Autodesk Fusion 360 part; units mm, degrees
(part 3 of 7)
  line L27 (11.5064, 2.3612) -> (11.4015, 2.3397)
  arc A55 (11.049, 2.5657) -> (11.4015, 2.3397) centre (11.3412, 2.6336) ccw
  arc A56 (11.049, 2.5657) -> (10.9184, 3.0745) centre (0, 0) ccw
  arc A57 (11.1184, 3.4424) -> (10.9184, 3.0745) centre (11.2071, 3.1559) ccw
  line L28 (11.1184, 3.4424) -> (11.2206, 3.4741)
  spline S28 degree 5 poles (11.2206, 3.4741) (11.2255, 3.4756) (11.2353, 3.4787) (11.2497, 3.4838) (11.2687, 3.4912) (11.2922, 3.5015) (11.3154, 3.5123) (11.3384, 3.5237) (11.3614, 3.5352) (11.3844, 3.5469) (11.4073, 3.5588) (11.4301, 3.5708) (11.4528, 3.5832) (11.4754, 3.5958) (11.4979, 3.6088) (11.5202, 3.6221) (11.5425, 3.6356) (11.5646, 3.6494) (11.5868, 3.6633) (11.6088, 3.6774) (11.6307, 3.6917) (11.6526, 3.7062) (11.6744, 3.7209) (11.6962, 3.7358) (11.7178, 3.7508) (11.7394, 3.7661) (11.7609, 3.7815) (11.7823, 3.7972) (11.8036, 3.8129) (11.8249, 3.8289) (11.8461, 3.845) (11.8672, 3.8612) (11.8883, 3.8777) (11.9093, 3.8942) (11.9302, 3.911) (11.9511, 3.9279) (11.9719, 3.9449) (11.9926, 3.9621) (12.0132, 3.9794) (12.0338, 3.9969) (12.0543, 4.0145) (12.0748, 4.0323) (12.0951, 4.0502) (12.1154, 4.0682) (12.1357, 4.0864) (12.1558, 4.1047) (12.1759, 4.1231) (12.196, 4.1417) (12.216, 4.1604) (12.2359, 4.1793) (12.2557, 4.1982) (12.2755, 4.2173) (12.2952, 4.2365) (12.3148, 4.2559) (12.3344, 4.2753) (12.3539, 4.2949) (12.3733, 4.3147) (12.3927, 4.3345) (12.412, 4.3544) (12.4313, 4.3745) (12.4504, 4.3947) (12.4695, 4.415) (12.4886, 4.4355) (12.5076, 4.456) (12.5265, 4.4767) (12.5453, 4.4974) (12.5641, 4.5183) (12.5828, 4.5393) (12.6015, 4.5604) (12.62, 4.5816) (12.6385, 4.603) (12.6533, 4.6201) (12.6643, 4.633) (12.6717, 4.6417) (12.6754, 4.646) knots 0 0 0 0 0 0 0.01428571 0.02857143 0.04285714 0.05714286 0.07142857 0.08571429 0.1 0.11428571 0.12857143 0.14285714 0.15714286 0.17142857 0.18571429 0.2 0.21428571 0.22857143 0.24285714 0.25714286 0.27142857 0.28571429 0.3 0.31428571 0.32857143 0.34285714 0.35714286 0.37142857 0.38571429 0.4 0.41428571 0.42857143 0.44285714 0.45714286 0.47142857 0.48571429 0.5 0.51428571 0.52857143 0.54285714 0.55714286 0.57142857 0.58571429 0.6 0.61428571 0.62857143 0.64285714 0.65714286 0.67142857 0.68571429 0.7 0.71428571 0.72857143 0.74285714 0.75714286 0.77142857 0.78571429 0.8 0.81428571 0.82857143 0.84285714 0.85714286 0.87142857 0.88571429 0.9 0.91428571 0.92857143 0.94285714 0.95714286 0.97142857 0.98571429 1 1 1 1 1 1
  arc A58 (12.6754, 4.646) -> (12.4203, 5.2901) centre (0, 0) ccw
  spline S29 degree 5 poles (12.4203, 5.2901) (12.4147, 5.2907) (12.4034, 5.292) (12.3866, 5.2939) (12.3641, 5.2963) (12.336, 5.2991) (12.3079, 5.3019) (12.2798, 5.3045) (12.2518, 5.307) (12.2238, 5.3094) (12.1959, 5.3116) (12.168, 5.3137) (12.1401, 5.3157) (12.1122, 5.3176) (12.0844, 5.3193) (12.0566, 5.3209) (12.0288, 5.3224) (12.0011, 5.3237) (11.9734, 5.3249) (11.9457, 5.3259) (11.9181, 5.3269) (11.8905, 5.3277) (11.8629, 5.3283) (11.8354, 5.3288) (11.8079, 5.3292) (11.7805, 5.3295) (11.7531, 5.3296) (11.7257, 5.3295) (11.6984, 5.3294) (11.6711, 5.3291) (11.6438, 5.3286) (11.6166, 5.328) (11.5895, 5.3272) (11.5624, 5.3263) (11.5353, 5.3253) (11.5083, 5.3241) (11.4814, 5.3227) (11.4544, 5.3212) (11.4276, 5.3196) (11.4008, 5.3178) (11.374, 5.3158) (11.3473, 5.3137) (11.3206, 5.3114) (11.2941, 5.309) (11.2675, 5.3064) (11.241, 5.3036) (11.2146, 5.3006) (11.1883, 5.2975) (11.1619, 5.2942) (11.1357, 5.2908) (11.1095, 5.2872) (11.0834, 5.2833) (11.0574, 5.2793) (11.0315, 5.2751) (11.0056, 5.2706) (10.9798, 5.266) (10.9541, 5.2612) (10.9284, 5.2563) (10.9029, 5.2511) (10.8774, 5.2458) (10.852, 5.2401) (10.8267, 5.2342) (10.8016, 5.228) (10.7766, 5.2214) (10.7517, 5.2146) (10.7269, 5.2076) (10.7021, 5.2004) (10.6775, 5.1931) (10.6529, 5.1855) (10.6285, 5.1776) (10.6045, 5.169) (10.5855, 5.1614) (10.5715, 5.1552) (10.5623, 5.1508) (10.5577, 5.1486) knots -1 -1 -1 -1 -1 -1 -0.98571429 -0.97142857 -0.95714286 -0.94285714 -0.92857143 -0.91428571 -0.9 -0.88571429 -0.87142857 -0.85714286 -0.84285714 -0.82857143 -0.81428571 -0.8 -0.78571429 -0.77142857 -0.75714286 -0.74285714 -0.72857143 -0.71428571 -0.7 -0.68571429 -0.67142857 -0.65714286 -0.64285714 -0.62857143 -0.61428571 -0.6 -0.58571429 -0.57142857 -0.55714286 -0.54285714 -0.52857143 -0.51428571 -0.5 -0.48571429 -0.47142857 -0.45714286 -0.44285714 -0.42857143 -0.41428571 -0.4 -0.38571429 -0.37142857 -0.35714286 -0.34285714 -0.32857143 -0.31428571 -0.3 -0.28571429 -0.27142857 -0.25714286 -0.24285714 -0.22857143 -0.21428571 -0.2 -0.18571429 -0.17142857 -0.15714286 -0.14285714 -0.12857143 -0.11428571 -0.1 -0.08571429 -0.07142857 -0.05714286 -0.04285714 -0.02857143 -0.01428571 0 0 0 0 0 0
  line L29 (10.5577, 5.1486) -> (10.4615, 5.1017)
  arc A59 (10.0638, 5.2329) -> (10.4615, 5.1017) centre (10.33, 5.3713) ccw
  arc A60 (10.0638, 5.2329) -> (9.8107, 5.6932) centre (0, 0) ccw
  arc A61 (9.913, 6.0993) -> (9.8107, 5.6932) centre (10.0702, 5.8438) ccw
  line L30 (9.913, 6.0993) -> (10.0042, 6.1554)
  spline S30 degree 5 poles (10.0042, 6.1554) (10.0085, 6.1581) (10.0171, 6.1635) (10.0299, 6.172) (10.0465, 6.184) (10.0666, 6.1997) (10.0864, 6.216) (10.1059, 6.2327) (10.1253, 6.2496) (10.1446, 6.2666) (10.1638, 6.2838) (10.1829, 6.3012) (10.2019, 6.3188) (10.2206, 6.3367) (10.2392, 6.3548) (10.2575, 6.3732) (10.2757, 6.3919) (10.2938, 6.4107) (10.3117, 6.4297) (10.3295, 6.4489) (10.3472, 6.4682) (10.3648, 6.4877) (10.3823, 6.5073) (10.3997, 6.5271) (10.4169, 6.5471) (10.434, 6.5672) (10.4509, 6.5875) (10.4678, 6.608) (10.4846, 6.6286) (10.5012, 6.6493) (10.5177, 6.6702) (10.5342, 6.6912) (10.5505, 6.7123) (10.5667, 6.7336) (10.5828, 6.755) (10.5988, 6.7766) (10.6147, 6.7982) (10.6305, 6.82) (10.6462, 6.842) (10.6617, 6.864) (10.6772, 6.8862) (10.6926, 6.9085) (10.7079, 6.9309) (10.7231, 6.9534) (10.7382, 6.976) (10.7531, 6.9988) (10.768, 7.0216) (10.7828, 7.0446) (10.7975, 7.0677) (10.8121, 7.0909) (10.8266, 7.1142) (10.841, 7.1376) (10.8553, 7.1611) (10.8695, 7.1847) (10.8836, 7.2085) (10.8977, 7.2323) (10.9116, 7.2562) (10.9254, 7.2803) (10.9392, 7.3044) (10.9528, 7.3286) (10.9664, 7.3529) (10.9798, 7.3774) (10.9932, 7.4019) (11.0065, 7.4265) (11.0196, 7.4512) (11.0327, 7.476) (11.0457, 7.5009) (11.0586, 7.5259) (11.0714, 7.551) (11.0841, 7.5762) (11.0968, 7.6014) (11.1068, 7.6217) (11.1143, 7.637) (11.1192, 7.6472) (11.1217, 7.6523) knots 0 0 0 0 0 0 0.01428571 0.02857143 0.04285714 0.05714286 0.07142857 0.08571429 0.1 0.11428571 0.12857143 0.14285714 0.15714286 0.17142857 0.18571429 0.2 0.21428571 0.22857143 0.24285714 0.25714286 0.27142857 0.28571429 0.3 0.31428571 0.32857143 0.34285714 0.35714286 0.37142857 0.38571429 0.4 0.41428571 0.42857143 0.44285714 0.45714286 0.47142857 0.48571429 0.5 0.51428571 0.52857143 0.54285714 0.55714286 0.57142857 0.58571429 0.6 0.61428571 0.62857143 0.64285714 0.65714286 0.67142857 0.68571429 0.7 0.71428571 0.72857143 0.74285714 0.75714286 0.77142857 0.78571429 0.8 0.81428571 0.82857143 0.84285714 0.85714286 0.87142857 0.88571429 0.9 0.91428571 0.92857143 0.94285714 0.95714286 0.97142857 0.98571429 1 1 1 1 1 1
  arc A62 (11.1217, 7.6523) -> (10.7145, 8.2127) centre (0, 0) ccw
  spline S31 degree 5 poles (10.7145, 8.2127) (10.7089, 8.2119) (10.6977, 8.2103) (10.6809, 8.2079) (10.6585, 8.2047) (10.6306, 8.2005) (10.6027, 8.1962) (10.5749, 8.1917) (10.5471, 8.1872) (10.5194, 8.1825) (10.4918, 8.1777) (10.4642, 8.1728) (10.4367, 8.1678) (10.4092, 8.1627) (10.3819, 8.1574) (10.3545, 8.1521) (10.3273, 8.1466) (10.3001, 8.141) (10.2729, 8.1352) (10.2459, 8.1294) (10.2189, 8.1234) (10.192, 8.1173) (10.1651, 8.1111) (10.1383, 8.1048) (10.1116, 8.0983) (10.085, 8.0917) (10.0584, 8.085) (10.0319, 8.0782) (10.0055, 8.0712) (9.9791, 8.0641) (9.9529, 8.0569) (9.9267, 8.0495) (9.9006, 8.0421) (9.8745, 8.0344) (9.8486, 8.0267) (9.8227, 8.0188) (9.7969, 8.0108) (9.7712, 8.0027) (9.7456, 7.9944) (9.7201, 7.986) (9.6947, 7.9774) (9.6693, 7.9687) (9.6441, 7.9599) (9.6189, 7.9509) (9.5939, 7.9418) (9.5689, 7.9325) (9.5441, 7.9231) (9.5193, 7.9135) (9.4947, 7.9038) (9.4701, 7.8939) (9.4457, 7.8839) (9.4213, 7.8737) (9.3971, 7.8633) (9.3731, 7.8527) (9.3491, 7.842) (9.3253, 7.8311) (9.3015, 7.8201) (9.2779, 7.8089) (9.2544, 7.7976) (9.2311, 7.786) (9.2079, 7.7743) (9.1849, 7.7623) (9.1621, 7.75) (9.1395, 7.7374) (9.1171, 7.7246) (9.0948, 7.7116) (9.0726, 7.6985) (9.0506, 7.6853) (9.0287, 7.6719) (9.007, 7.6581) (8.9858, 7.6438) (8.9694, 7.6317) (8.9573, 7.6222) (8.9495, 7.6157) (8.9456, 7.6124) knots -1 -1 -1 -1 -1 -1 -0.98571429 -0.97142857 -0.95714286 -0.94285714 -0.92857143 -0.91428571 -0.9 -0.88571429 -0.87142857 -0.85714286 -0.84285714 -0.82857143 -0.81428571 -0.8 -0.78571429 -0.77142857 -0.75714286 -0.74285714 -0.72857143 -0.71428571 -0.7 -0.68571429 -0.67142857 -0.65714286 -0.64285714 -0.62857143 -0.61428571 -0.6 -0.58571429 -0.57142857 -0.55714286 -0.54285714 -0.52857143 -0.51428571 -0.5 -0.48571429 -0.47142857 -0.45714286 -0.44285714 -0.42857143 -0.41428571 -0.4 -0.38571429 -0.37142857 -0.35714286 -0.34285714 -0.32857143 -0.31428571 -0.3 -0.28571429 -0.27142857 -0.25714286 -0.24285714 -0.22857143 -0.21428571 -0.2 -0.18571429 -0.17142857 -0.15714286 -0.14285714 -0.12857143 -0.11428571 -0.1 -0.08571429 -0.07142857 -0.05714286 -0.04285714 -0.02857143 -0.01428571 0 0 0 0 0 0
  line L31 (8.9456, 7.6124) -> (8.8641, 7.543)
  arc A63 (8.4463, 7.5713) -> (8.8641, 7.543) centre (8.6697, 7.7715) ccw
  arc A64 (8.4463, 7.5713) -> (8.0867, 7.9542) centre (0, 0) ccw
  arc A65 (8.0847, 8.373) -> (8.0867, 7.9542) centre (8.3005, 8.1646) ccw
  line L32 (8.0847, 8.373) -> (8.1591, 8.45)
  spline S32 degree 5 poles (8.1591, 8.45) (8.1626, 8.4536) (8.1696, 8.4611) (8.1799, 8.4725) (8.1929, 8.4881) (8.2086, 8.5084) (8.2237, 8.5291) (8.2384, 8.5501) (8.253, 8.5713) (8.2675, 8.5926) (8.2818, 8.6141) (8.296, 8.6356) (8.31, 8.6574) (8.3237, 8.6793) (8.3371, 8.7015) (8.3503, 8.724) (8.3633, 8.7465) (8.3761, 8.7693) (8.3887, 8.7922) (8.4012, 8.8151) (8.4136, 8.8383) (8.4258, 8.8615) (8.4378, 8.8848) (8.4497, 8.9083) (8.4614, 8.932) (8.473, 8.9557) (8.4844, 8.9796) (8.4956, 9.0036) (8.5067, 9.0277) (8.5177, 9.052) (8.5285, 9.0763) (8.5392, 9.1007) (8.5497, 9.1253) (8.5601, 9.1499) (8.5704, 9.1746) (8.5806, 9.1995) (8.5906, 9.2244) (8.6004, 9.2495) (8.6102, 9.2746) (8.6198, 9.2998) (8.6293, 9.3252) (8.6386, 9.3506) (8.6479, 9.3761) (8.657, 9.4017) (8.6659, 9.4273) (8.6748, 9.4531) (8.6835, 9.4789) (8.6921, 9.5049) (8.7006, 9.5309) (8.709, 9.557) (8.7172, 9.5832) (8.7254, 9.6094) (8.7334, 9.6357) (8.7413, 9.6622) (8.749, 9.6887) (8.7567, 9.7152) (8.7642, 9.7419) (8.7717, 9.7686) (8.779, 9.7954) (8.7862, 9.8222) (8.7932, 9.8492) (8.8002, 9.8762) (8.807, 9.9032) (8.8138, 9.9304) (8.8204, 9.9576) (8.8269, 9.9849) (8.8333, 10.0122) (8.8396, 10.0396) (8.8457, 10.0671) (8.8518, 10.0947) (8.8577, 10.1223) (8.8624, 10.1444) (8.8659, 10.1611) (8.8681, 10.1722) (8.8693, 10.1777) knots 0 0 0 0 0 0 0.01428571 0.02857143 0.04285714 0.05714286 0.07142857 0.08571429 0.1 0.11428571 0.12857143 0.14285714 0.15714286 0.17142857 0.18571429 0.2 0.21428571 0.22857143 0.24285714 0.25714286 0.27142857 0.28571429 0.3 0.31428571 0.32857143 0.34285714 0.35714286 0.37142857 0.38571429 0.4 0.41428571 0.42857143 0.44285714 0.45714286 0.47142857 0.48571429 0.5 0.51428571 0.52857143 0.54285714 0.55714286 0.57142857 0.58571429 0.6 0.61428571 0.62857143 0.64285714 0.65714286 0.67142857 0.68571429 0.7 0.71428571 0.72857143 0.74285714 0.75714286 0.77142857 0.78571429 0.8 0.81428571 0.82857143 0.84285714 0.85714286 0.87142857 0.88571429 0.9 0.91428571 0.92857143 0.94285714 0.95714286 0.97142857 0.98571429 1 1 1 1 1 1
  arc A66 (8.8693, 10.1777) -> (8.3355, 10.6193) centre (0, 0) ccw
  spline S33 degree 5 poles (8.3355, 10.6193) (8.3303, 10.6171) (8.3198, 10.6128) (8.3041, 10.6063) (8.2832, 10.5976) (8.2572, 10.5866) (8.2313, 10.5754) (8.2054, 10.5642) (8.1797, 10.5529) (8.154, 10.5415) (8.1284, 10.53) (8.103, 10.5184) (8.0776, 10.5067) (8.0522, 10.4949) (8.027, 10.483) (8.0019, 10.471) (7.9768, 10.4589) (7.9519, 10.4467) (7.9271, 10.4344) (7.9023, 10.422) (7.8776, 10.4095) (7.8531, 10.3969) (7.8286, 10.3842) (7.8042, 10.3714) (7.78, 10.3585) (7.7558, 10.3455) (7.7317, 10.3324) (7.7078, 10.3192) (7.6839, 10.3059) (7.6602, 10.2925) (7.6365, 10.2789) (7.613, 10.2653) (7.5895, 10.2516) (7.5662, 10.2377) (7.543, 10.2238) (7.5199, 10.2097) (7.4969, 10.1955) (7.4741, 10.1813) (7.4513, 10.1669) (7.4287, 10.1524) (7.4062, 10.1378) (7.3838, 10.123) (7.3616, 10.1082) (7.3394, 10.0932) (7.3174, 10.0782) (7.2956, 10.063) (7.2738, 10.0477) (7.2522, 10.0322) (7.2308, 10.0167) (7.2094, 10.001) (7.1883, 9.9852) (7.1672, 9.9693) (7.1464, 9.9532) (7.1257, 9.937) (7.1052, 9.9207) (7.0848, 9.9042) (7.0645, 9.8876) (7.0444, 9.8709) (7.0245, 9.8541) (7.0047, 9.8371) (6.9852, 9.8199) (6.9659, 9.8026) (6.9469, 9.785) (6.9281, 9.7672) (6.9096, 9.7492) (6.8913, 9.7311) (6.8731, 9.7129) (6.855, 9.6946) (6.8371, 9.6762) (6.8196, 9.6575) (6.8026, 9.6383) (6.7896, 9.6225) (6.7804, 9.6104) (6.7744, 9.6021) (6.7714, 9.5979) knots -1 -1 -1 -1 -1 -1 -0.98571429 -0.97142857 -0.95714286 -0.94285714 -0.92857143 -0.91428571 -0.9 -0.88571429 -0.87142857 -0.85714286 -0.84285714 -0.82857143 -0.81428571 -0.8 -0.78571429 -0.77142857 -0.75714286 -0.74285714 -0.72857143 -0.71428571 -0.7 -0.68571429 -0.67142857 -0.65714286 -0.64285714 -0.62857143 -0.61428571 -0.6 -0.58571429 -0.57142857 -0.55714286 -0.54285714 -0.52857143 -0.51428571 -0.5 -0.48571429 -0.47142857 -0.45714286 -0.44285714 -0.42857143 -0.41428571 -0.4 -0.38571429 -0.37142857 -0.35714286 -0.34285714 -0.32857143 -0.31428571 -0.3 -0.28571429 -0.27142857 -0.25714286 -0.24285714 -0.22857143 -0.21428571 -0.2 -0.18571429 -0.17142857 -0.15714286 -0.14285714 -0.12857143 -0.11428571 -0.1 -0.08571429 -0.07142857 -0.05714286 -0.04285714 -0.02857143 -0.01428571 0 0 0 0 0 0
  line L33 (6.7714, 9.5979) -> (6.7097, 9.5105)
  arc A67 (6.298, 9.4339) -> (6.7097, 9.5105) centre (6.4646, 9.6834) ccw
  arc A68 (6.298, 9.4339) -> (5.8545, 9.7154) centre (0, 0) ccw
  arc A69 (5.7485, 10.1205) -> (5.8545, 9.7154) centre (6.0093, 9.9723) ccw
  line L34 (5.7485, 10.1205) -> (5.8013, 10.2136)
  spline S34 degree 5 poles (5.8013, 10.2136) (5.8038, 10.218) (5.8088, 10.2269) (5.8159, 10.2405) (5.8246, 10.259) (5.8347, 10.2825) (5.8442, 10.3063) (5.8533, 10.3303) (5.8621, 10.3545) (5.8708, 10.3787) (5.8794, 10.403) (5.8878, 10.4274) (5.8959, 10.452) (5.9037, 10.4767) (5.9112, 10.5015) (5.9184, 10.5265) (5.9254, 10.5516) (5.9321, 10.5768) (5.9387, 10.6021) (5.9451, 10.6275) (5.9513, 10.653) (5.9573, 10.6785) (5.9632, 10.7041) (5.9688, 10.7298) (5.9743, 10.7556) (5.9796, 10.7815) (5.9847, 10.8075) (5.9896, 10.8335) (5.9943, 10.8597) (5.9989, 10.8858) (6.0034, 10.9121) (6.0077, 10.9384) (6.0118, 10.9648) (6.0157, 10.9913) (6.0195, 11.0178) (6.0232, 11.0444) (6.0266, 11.071) (6.03, 11.0977) (6.0332, 11.1245) (6.0362, 11.1513) (6.0391, 11.1782) (6.0418, 11.2051) (6.0444, 11.2321) (6.0469, 11.2592) (6.0492, 11.2863) (6.0514, 11.3134) (6.0534, 11.3406) (6.0553, 11.3679) (6.057, 11.3952) (6.0587, 11.4226) (6.0601, 11.45) (6.0615, 11.4774) (6.0627, 11.5049) (6.0638, 11.5325) (6.0647, 11.5601) (6.0655, 11.5877) (6.0662, 11.6154) (6.0667, 11.6431) (6.0671, 11.6709) (6.0674, 11.6987) (6.0676, 11.7265) (6.0676, 11.7544) (6.0675, 11.7823) (6.0673, 11.8103) (6.0669, 11.8383) (6.0664, 11.8663) (6.0658, 11.8944) (6.0651, 11.9225) (6.0642, 11.9507) (6.0633, 11.9789) (6.0622, 12.0071) (6.0612, 12.0297) (6.0604, 12.0467) (6.0598, 12.058) (6.0595, 12.0637) knots 0 0 0 0 0 0 0.01428571 0.02857143 0.04285714 0.05714286 0.07142857 0.08571429 0.1 0.11428571 0.12857143 0.14285714 0.15714286 0.17142857 0.18571429 0.2 0.21428571 0.22857143 0.24285714 0.25714286 0.27142857 0.28571429 0.3 0.31428571 0.32857143 0.34285714 0.35714286 0.37142857 0.38571429 0.4 0.41428571 0.42857143 0.44285714 0.45714286 0.47142857 0.48571429 0.5 0.51428571 0.52857143 0.54285714 0.55714286 0.57142857 0.58571429 0.6 0.61428571 0.62857143 0.64285714 0.65714286 0.67142857 0.68571429 0.7 0.71428571 0.72857143 0.74285714 0.75714286 0.77142857 0.78571429 0.8 0.81428571 0.82857143 0.84285714 0.85714286 0.87142857 0.88571429 0.9 0.91428571 0.92857143 0.94285714 0.95714286 0.97142857 0.98571429 1 1 1 1 1 1
  arc A70 (6.0595, 12.0637) -> (5.4327, 12.3586) centre (0, 0) ccw
  spline S35 degree 5 poles (5.4327, 12.3586) (5.4282, 12.3552) (5.4191, 12.3484) (5.4055, 12.3382) (5.3875, 12.3246) (5.365, 12.3074) (5.3427, 12.2902) (5.3204, 12.273) (5.2983, 12.2556) (5.2763, 12.2382) (5.2544, 12.2207) (5.2326, 12.2031) (5.2109, 12.1854) (5.1893, 12.1677) (5.1678, 12.1499) (5.1465, 12.1321) (5.1252, 12.1141) (5.1041, 12.0961) (5.0831, 12.078) (5.0622, 12.0598) (5.0414, 12.0416) (5.0207, 12.0233) (5.0002, 12.0049) (4.9798, 11.9864) (4.9595, 11.9679) (4.9393, 11.9493) (4.9193, 11.9306) (4.8993, 11.9119) (4.8795, 11.893) (4.8599, 11.8741) (4.8403, 11.8551) (4.8209, 11.8361) (4.8016, 11.8169) (4.7825, 11.7977) (4.7635, 11.7784) (4.7446, 11.7591) (4.7259, 11.7396) (4.7073, 11.7201) (4.6888, 11.7005) (4.6705, 11.6809) (4.6524, 11.6611) (4.6343, 11.6413) (4.6165, 11.6214) (4.5988, 11.6014) (4.5812, 11.5813) (4.5638, 11.5612) (4.5466, 11.5409) (4.5295, 11.5206) (4.5126, 11.5002) (4.4958, 11.4797) (4.4792, 11.4592) (4.4628, 11.4385) (4.4466, 11.4178) (4.4306, 11.3969) (4.4148, 11.376) (4.3991, 11.355) (4.3836, 11.3339) (4.3683, 11.3127) (4.3532, 11.2914) (4.3383, 11.2701) (4.3236, 11.2486) (4.3093, 11.227) (4.2952, 11.2052) (4.2815, 11.1833) (4.268, 11.1613) (4.2547, 11.1392) (4.2416, 11.117) (4.2287, 11.0948) (4.2159, 11.0725) (4.2036, 11.05) (4.1919, 11.0273) (4.1833, 11.0088) (4.1773, 10.9946) (4.1736, 10.9851) (4.1718, 10.9804) knots -1 -1 -1 -1 -1 -1 -0.98571429 -0.97142857 -0.95714286 -0.94285714 -0.92857143 -0.91428571 -0.9 -0.88571429 -0.87142857 -0.85714286 -0.84285714 -0.82857143 -0.81428571 -0.8 -0.78571429 -0.77142857 -0.75714286 -0.74285714 -0.72857143 -0.71428571 -0.7 -0.68571429 -0.67142857 -0.65714286 -0.64285714 -0.62857143 -0.61428571 -0.6 -0.58571429 -0.57142857 -0.55714286 -0.54285714 -0.52857143 -0.51428571 -0.5 -0.48571429 -0.47142857 -0.45714286 -0.44285714 -0.42857143 -0.41428571 -0.4 -0.38571429 -0.37142857 -0.35714286 -0.34285714 -0.32857143 -0.31428571 -0.3 -0.28571429 -0.27142857 -0.25714286 -0.24285714 -0.22857143 -0.21428571 -0.2 -0.18571429 -0.17142857 -0.15714286 -0.14285714 -0.12857143 -0.11428571 -0.1 -0.08571429 -0.07142857 -0.05714286 -0.04285714 -0.02857143 -0.01428571 0 0 0 0 0 0
  line L35 (4.1718, 10.9804) -> (4.1338, 10.8803)
  arc A71 (3.754, 10.7038) -> (4.1338, 10.8803) centre (3.8533, 10.9869) ccw
  arc A72 (3.754, 10.7038) -> (3.2544, 10.8661) centre (0, 0) ccw
  arc A73 (3.051, 11.2321) -> (3.2544, 10.8661) centre (3.3405, 11.1535) ccw
  line L36 (3.051, 11.2321) -> (3.0791, 11.3354)
  spline S36 degree 5 poles (3.0791, 11.3354) (3.0804, 11.3403) (3.083, 11.3502) (3.0864, 11.3652) (3.0903, 11.3852) (3.0943, 11.4105) (3.0975, 11.4359) (3.1003, 11.4614) (3.1029, 11.487) (3.1053, 11.5127) (3.1075, 11.5383) (3.1096, 11.5641) (3.1113, 11.5899) (3.1128, 11.6157) (3.1139, 11.6417) (3.1146, 11.6676) (3.1151, 11.6937) (3.1154, 11.7198) (3.1154, 11.7459) (3.1153, 11.7721) (3.115, 11.7983) (3.1145, 11.8245) (3.1138, 11.8508) (3.1129, 11.8771) (3.1118, 11.9035) (3.1105, 11.9299) (3.1089, 11.9563) (3.1072, 11.9827) (3.1053, 12.0092) (3.1033, 12.0357) (3.101, 12.0622) (3.0986, 12.0888) (3.0961, 12.1154) (3.0933, 12.142) (3.0904, 12.1686) (3.0873, 12.1953) (3.0841, 12.222) (3.0806, 12.2487) (3.0771, 12.2754) (3.0733, 12.3021) (3.0695, 12.3289) (3.0654, 12.3556) (3.0612, 12.3824) (3.0569, 12.4093) (3.0524, 12.4361) (3.0477, 12.4629) (3.0429, 12.4898) (3.038, 12.5167) (3.0329, 12.5435) (3.0276, 12.5704) (3.0223, 12.5973) (3.0167, 12.6243) (3.0111, 12.6512) (3.0053, 12.6782) (2.9993, 12.7051) (2.9932, 12.7321) (2.987, 12.7591) (2.9806, 12.786) (2.9741, 12.813) (2.9675, 12.84) (2.9607, 12.8671) (2.9538, 12.8941) (2.9467, 12.9211) (2.9396, 12.9481) (2.9323, 12.9752) (2.9248, 13.0022) (2.9172, 13.0293) (2.9095, 13.0563) (2.9017, 13.0834) (2.8937, 13.1104) (2.8857, 13.1375) (2.8791, 13.1591) (2.8741, 13.1754) (2.8707, 13.1862) (2.8691, 13.1916) knots 0 0 0 0 0 0 0.01428571 0.02857143 0.04285714 0.05714286 0.07142857 0.08571429 0.1 0.11428571 0.12857143 0.14285714 0.15714286 0.17142857 0.18571429 0.2 0.21428571 0.22857143 0.24285714 0.25714286 0.27142857 0.28571429 0.3 0.31428571 0.32857143 0.34285714 0.35714286 0.37142857 0.38571429 0.4 0.41428571 0.42857143 0.44285714 0.45714286 0.47142857 0.48571429 0.5 0.51428571 0.52857143 0.54285714 0.55714286 0.57142857 0.58571429 0.6 0.61428571 0.62857143 0.64285714 0.65714286 0.67142857 0.68571429 0.7 0.71428571 0.72857143 0.74285714 0.75714286 0.77142857 0.78571429 0.8 0.81428571 0.82857143 0.84285714 0.85714286 0.87142857 0.88571429 0.9 0.91428571 0.92857143 0.94285714 0.95714286 0.97142857 0.98571429 1 1 1 1 1 1
  arc A74 (2.8691, 13.1916) -> (2.1886, 13.3214) centre (0, 0) ccw
  spline S37 degree 5 poles (2.1886, 13.3214) (2.185, 13.317) (2.1779, 13.3082) (2.1673, 13.2949) (2.1532, 13.2772) (2.1357, 13.255) (2.1184, 13.2328) (2.1011, 13.2105) (2.084, 13.1882) (2.067, 13.1658) (2.0501, 13.1434) (2.0334, 13.121) (2.0168, 13.0985) (2.0003, 13.076) (1.9839, 13.0534) (1.9677, 13.0308) (1.9515, 13.0081) (1.9356, 12.9854) (1.9197, 12.9627) (1.904, 12.9399) (1.8884, 12.917) (1.8729, 12.8942) (1.8576, 12.8712) (1.8424, 12.8483) (1.8274, 12.8253) (1.8125, 12.8022) (1.7977, 12.7792) (1.7831, 12.756) (1.7686, 12.7329) (1.7542, 12.7097) (1.74, 12.6864) (1.7259, 12.6631) (1.712, 12.6398) (1.6983, 12.6164) (1.6847, 12.593) (1.6712, 12.5696) (1.6579, 12.5461) (1.6447, 12.5226) (1.6317, 12.499) (1.6189, 12.4754) (1.6062, 12.4518) (1.5937, 12.4281) (1.5813, 12.4043) (1.5691, 12.3806) (1.5571, 12.3568) (1.5453, 12.3329) (1.5336, 12.309) (1.5221, 12.2851) (1.5108, 12.2611) (1.4997, 12.2371) (1.4887, 12.2131) (1.478, 12.189) (1.4674, 12.1649) (1.4571, 12.1407) (1.447, 12.1165) (1.437, 12.0922) (1.4273, 12.068) (1.4177, 12.0436) (1.4084, 12.0193) (1.3992, 11.9949) (1.3904, 11.9704) (1.3819, 11.9459) (1.3737, 11.9213) (1.3658, 11.8967) (1.3582, 11.872) (1.3509, 11.8473) (1.3437, 11.8226) (1.3366, 11.7979) (1.3298, 11.7731) (1.3235, 11.7483) (1.3178, 11.7233) (1.3141, 11.7032) (1.3118, 11.6881) (1.3106, 11.678) (1.31, 11.6729) knots -1 -1 -1 -1 -1 -1 -0.98571429 -0.97142857 -0.95714286 -0.94285714 -0.92857143 -0.91428571 -0.9 -0.88571429 -0.87142857 -0.85714286 -0.84285714 -0.82857143 -0.81428571 -0.8 -0.78571429 -0.77142857 -0.75714286 -0.74285714 -0.72857143 -0.71428571 -0.7 -0.68571429 -0.67142857 -0.65714286 -0.64285714 -0.62857143 -0.61428571 -0.6 -0.58571429 -0.57142857 -0.55714286 -0.54285714 -0.52857143 -0.51428571 -0.5 -0.48571429 -0.47142857 -0.45714286 -0.44285714 -0.42857143 -0.41428571 -0.4 -0.38571429 -0.37142857 -0.35714286 -0.34285714 -0.32857143 -0.31428571 -0.3 -0.28571429 -0.27142857 -0.25714286 -0.24285714 -0.22857143 -0.21428571 -0.2 -0.18571429 -0.17142857 -0.15714286 -0.14285714 -0.12857143 -0.11428571 -0.1 -0.08571429 -0.07142857 -0.05714286 -0.04285714 -0.02857143 -0.01428571 0 0 0 0 0 0
  line L37 (1.31, 11.6729) -> (1.2981, 11.5665)
  arc A75 (0.9742, 11.3011) -> (1.2981, 11.5665) centre (0.9999, 11.6) ccw
  arc A76 (0.9742, 11.3011) -> (0.4499, 11.3341) centre (0, 0) ccw
  arc A77 (0.1618, 11.638) -> (0.4499, 11.3341) centre (0.4618, 11.6338) ccw
  line L38 (0.1618, 11.638) -> (0.1633, 11.745)
  spline S38 degree 5 poles (0.1633, 11.745) (0.1634, 11.7501) (0.1634, 11.7603) (0.1631, 11.7757) (0.1619, 11.796) (0.1594, 11.8215) (0.1562, 11.8469) (0.1526, 11.8724) (0.1487, 11.8978) (0.1447, 11.9232) (0.1404, 11.9487) (0.136, 11.9741) (0.1313, 11.9995) (0.1263, 12.0249) (0.1209, 12.0503) (0.1151, 12.0757) (0.1091, 12.101) (0.1029, 12.1264) (0.0965, 12.1517) (0.0899, 12.177) (0.083, 12.2023) (0.076, 12.2276) (0.0688, 12.2529) (0.0614, 12.2781) (0.0537, 12.3034) (0.0459, 12.3286) (0.0378, 12.3538) (0.0296, 12.379) (0.0212, 12.4042) (0.0126, 12.4293) (0.0039, 12.4545) (-0.0051, 12.4796) (-0.0142, 12.5047) (-0.0235, 12.5298) (-0.0329, 12.5549) (-0.0425, 12.5799) (-0.0523, 12.605) (-0.0623, 12.63) (-0.0724, 12.655) (-0.0826, 12.6799) (-0.093, 12.7049) (-0.1036, 12.7298) (-0.1143, 12.7547) (-0.1252, 12.7796) (-0.1363, 12.8045) (-0.1474, 12.8293) (-0.1588, 12.8541) (-0.1702, 12.8789) (-0.1819, 12.9037) (-0.1936, 12.9285) (-0.2055, 12.9532) (-0.2176, 12.9779) (-0.2298, 13.0026) (-0.2421, 13.0272) (-0.2546, 13.0519) (-0.2672, 13.0765) (-0.2799, 13.101) (-0.2928, 13.1256) (-0.3058, 13.1501) (-0.3189, 13.1746) (-0.3322, 13.1991) (-0.3456, 13.2236) (-0.3592, 13.248) (-0.3729, 13.2724) (-0.3867, 13.2967) (-0.4006, 13.3211) (-0.4147, 13.3454) (-0.4288, 13.3697) (-0.4432, 13.3939) (-0.4576, 13.4182) (-0.4722, 13.4424) (-0.4839, 13.4617) (-0.4928, 13.4762) (-0.4987, 13.4858) (-0.5017, 13.4907) knots 0 0 0 0 0 0 0.01428571 0.02857143 0.04285714 0.05714286 0.07142857 0.08571429 0.1 0.11428571 0.12857143 0.14285714 0.15714286 0.17142857 0.18571429 0.2 0.21428571 0.22857143 0.24285714 0.25714286 0.27142857 0.28571429 0.3 0.31428571 0.32857143 0.34285714 0.35714286 0.37142857 0.38571429 0.4 0.41428571 0.42857143 0.44285714 0.45714286 0.47142857 0.48571429 0.5 0.51428571 0.52857143 0.54285714 0.55714286 0.57142857 0.58571429 0.6 0.61428571 0.62857143 0.64285714 0.65714286 0.67142857 0.68571429 0.7 0.71428571 0.72857143 0.74285714 0.75714286 0.77142857 0.78571429 0.8 0.81428571 0.82857143 0.84285714 0.85714286 0.87142857 0.88571429 0.9 0.91428571 0.92857143 0.94285714 0.95714286 0.97142857 0.98571429 1 1 1 1 1 1
  arc A78 (-0.5017, 13.4907) -> (-1.1931, 13.4472) centre (0, 0) ccw
  spline S39 degree 5 poles (-1.1931, 13.4472) (-1.1954, 13.442) (-1.2001, 13.4317) (-1.2071, 13.4162) (-1.2163, 13.3956) (-1.2278, 13.3697) (-1.239, 13.3439) (-1.2502, 13.318) (-1.2612, 13.2921) (-1.2721, 13.2663) (-1.2829, 13.2404) (-1.2936, 13.2145) (-1.3041, 13.1885) (-1.3144, 13.1626) (-1.3247, 13.1367) (-1.3348, 13.1107) (-1.3448, 13.0848) (-1.3546, 13.0588) (-1.3643, 13.0328) (-1.3739, 13.0068) (-1.3833, 12.9808) (-1.3926, 12.9548) (-1.4017, 12.9288) (-1.4107, 12.9028) (-1.4196, 12.8768) (-1.4283, 12.8508) (-1.4368, 12.8247) (-1.4453, 12.7987) (-1.4535, 12.7727) (-1.4617, 12.7466) (-1.4696, 12.7206) (-1.4775, 12.6945) (-1.4851, 12.6685) (-1.4927, 12.6424) (-1.5, 12.6164) (-1.5072, 12.5903) (-1.5143, 12.5642) (-1.5212, 12.5382) (-1.5279, 12.5121) (-1.5345, 12.4861) (-1.5409, 12.46) (-1.5471, 12.4339) (-1.5532, 12.4079) (-1.5591, 12.3818) (-1.5648, 12.3558) (-1.5703, 12.3298) (-1.5757, 12.3037) (-1.5809, 12.2777) (-1.5859, 12.2517) (-1.5907, 12.2256) (-1.5953, 12.1996) (-1.5998, 12.1736) (-1.604, 12.1476) (-1.608, 12.1216) (-1.6117, 12.0957) (-1.6153, 12.0697) (-1.6187, 12.0438) (-1.6219, 12.0178) (-1.6249, 11.9919) (-1.6277, 11.966) (-1.6302, 11.9401) (-1.6324, 11.9143) (-1.6342, 11.8884) (-1.6357, 11.8626) (-1.6369, 11.8368) (-1.6379, 11.8111) (-1.6387, 11.7853) (-1.6394, 11.7596) (-1.6398, 11.7339) (-1.6398, 11.7083) (-1.639, 11.6827) (-1.6376, 11.6624) (-1.6361, 11.6471) (-1.6348, 11.637) (-1.6341, 11.6319) knots -1 -1 -1 -1 -1 -1 -0.98571429 -0.97142857 -0.95714286 -0.94285714 -0.92857143 -0.91428571 -0.9 -0.88571429 -0.87142857 -0.85714286 -0.84285714 -0.82857143 -0.81428571 -0.8 -0.78571429 -0.77142857 -0.75714286 -0.74285714 -0.72857143 -0.71428571 -0.7 -0.68571429 -0.67142857 -0.65714286 -0.64285714 -0.62857143 -0.61428571 -0.6 -0.58571429 -0.57142857 -0.55714286 -0.54285714 -0.52857143 -0.51428571 -0.5 -0.48571429 -0.47142857 -0.45714286 -0.44285714 -0.42857143 -0.41428571 -0.4 -0.38571429 -0.37142857 -0.35714286 -0.34285714 -0.32857143 -0.31428571 -0.3 -0.28571429 -0.27142857 -0.25714286 -0.24285714 -0.22857143 -0.21428571 -0.2 -0.18571429 -0.17142857 -0.15714286 -0.14285714 -0.12857143 -0.11428571 -0.1 -0.08571429 -0.07142857 -0.05714286 -0.04285714 -0.02857143 -0.01428571 0 0 0 0 0 0
  line L39 (-1.6341, 11.6319) -> (-1.6192, 11.526)
  arc A79 (-1.8669, 11.1883) -> (-1.6192, 11.526) centre (-1.9163, 11.4842) ccw
  arc A80 (-1.8669, 11.1883) -> (-2.3829, 11.0899) centre (0, 0) ccw
  arc A81 (-2.7375, 11.3126) -> (-2.3829, 11.0899) centre (-2.4459, 11.3832) ccw
  line L40 (-2.7375, 11.3126) -> (-2.7627, 11.4166)
  spline S40 degree 5 poles (-2.7627, 11.4166) (-2.7639, 11.4216) (-2.7664, 11.4315) (-2.7706, 11.4463) (-2.7768, 11.4657) (-2.7855, 11.4897) (-2.7949, 11.5136) (-2.8048, 11.5373) (-2.8148, 11.561) (-2.8251, 11.5846) (-2.8355, 11.6082) (-2.8461, 11.6317) (-2.857, 11.6552) (-2.8682, 11.6785) (-2.8797, 11.7018) (-2.8916, 11.7249) (-2.9037, 11.748) (-2.916, 11.771) (-2.9286, 11.7939) (-2.9413, 11.8168) (-2.9542, 11.8396) (-2.9672, 11.8624) (-2.9805, 11.885) (-2.994, 11.9077) (-3.0077, 11.9302) (-3.0215, 11.9527) (-3.0356, 11.9751) (-3.0499, 11.9975) (-3.0643, 12.0198) (-3.0788, 12.042) (-3.0936, 12.0642) (-3.1085, 12.0863) (-3.1235, 12.1083) (-3.1388, 12.1303) (-3.1541, 12.1523) (-3.1697, 12.1741) (-3.1854, 12.1959) (-3.2012, 12.2177) (-3.2172, 12.2394) (-3.2334, 12.261) (-3.2497, 12.2826) (-3.2661, 12.3041) (-3.2827, 12.3256) (-3.2994, 12.347) (-3.3163, 12.3683) (-3.3333, 12.3896) (-3.3505, 12.4108) (-3.3677, 12.432) (-3.3852, 12.4531) (-3.4027, 12.4741) (-3.4204, 12.4951) (-3.4382, 12.5161) (-3.4562, 12.5369) (-3.4742, 12.5577) (-3.4924, 12.5785) (-3.5108, 12.5992) (-3.5292, 12.6198) (-3.5478, 12.6404) (-3.5665, 12.6609) (-3.5853, 12.6814) (-3.6043, 12.7018) (-3.6233, 12.7222) (-3.6425, 12.7424) (-3.6618, 12.7627) (-3.6813, 12.7828) (-3.7008, 12.803) (-3.7205, 12.823) (-3.7403, 12.843) (-3.7602, 12.8629) (-3.7802, 12.8828) (-3.8003, 12.9026) (-3.8165, 12.9184) (-3.8287, 12.9303) (-3.8369, 12.9381) (-3.8409, 12.9421) knots 0 0 0 0 0 0 0.01428571 0.02857143 0.04285714 0.05714286 0.07142857 0.08571429 0.1 0.11428571 0.12857143 0.14285714 0.15714286 0.17142857 0.18571429 0.2 0.21428571 0.22857143 0.24285714 0.25714286 0.27142857 0.28571429 0.3 0.31428571 0.32857143 0.34285714 0.35714286 0.37142857 0.38571429 0.4 0.41428571 0.42857143 0.44285714 0.45714286 0.47142857 0.48571429 0.5 0.51428571 0.52857143 0.54285714 0.55714286 0.57142857 0.58571429 0.6 0.61428571 0.62857143 0.64285714 0.65714286 0.67142857 0.68571429 0.7 0.71428571 0.72857143 0.74285714 0.75714286 0.77142857 0.78571429 0.8 0.81428571 0.82857143 0.84285714 0.85714286 0.87142857 0.88571429 0.9 0.91428571 0.92857143 0.94285714 0.95714286 0.97142857 0.98571429 1 1 1 1 1 1
  arc A82 (-3.8409, 12.9421) -> (-4.4998, 12.728) centre (0, 0) ccw
  spline S41 degree 5 poles (-4.4998, 12.728) (-4.5008, 12.7224) (-4.5027, 12.7113) (-4.5056, 12.6945) (-4.5095, 12.6722) (-4.5141, 12.6444) (-4.5186, 12.6165) (-4.523, 12.5887) (-4.5272, 12.5609) (-4.5314, 12.5331) (-4.5354, 12.5053) (-4.5392, 12.4776) (-4.5429, 12.4499) (-4.5465, 12.4222) (-4.55, 12.3945) (-4.5534, 12.3669) (-4.5566, 12.3393) (-4.5596, 12.3117) (-4.5626, 12.2841) (-4.5654, 12.2565) (-4.568, 12.229) (-4.5705, 12.2015) (-4.5729, 12.1741) (-4.5752, 12.1466) (-4.5773, 12.1192) (-4.5793, 12.0919) (-4.5811, 12.0645) (-4.5828, 12.0372) (-4.5843, 12.0099) (-4.5857, 11.9827) (-4.587, 11.9555) (-4.5881, 11.9283) (-4.589, 11.9011) (-4.5898, 11.874) (-4.5905, 11.847) (-4.591, 11.8199) (-4.5913, 11.7929) (-4.5915, 11.766) (-4.5916, 11.7391) (-4.5914, 11.7122) (-4.5912, 11.6853) (-4.5907, 11.6586) (-4.5901, 11.6318) (-4.5893, 11.6051) (-4.5884, 11.5785) (-4.5873, 11.5519) (-4.586, 11.5253) (-4.5845, 11.4988) (-4.5829, 11.4724) (-4.5811, 11.446) (-4.5791, 11.4196) (-4.577, 11.3933) (-4.5746, 11.3671) (-4.572, 11.3409) (-4.5692, 11.3148) (-4.5662, 11.2888) (-4.563, 11.2628) (-4.5597, 11.2369) (-4.5562, 11.2111) (-4.5524, 11.1853) (-4.5484, 11.1596) (-4.5441, 11.134) (-4.5394, 11.1085) (-4.5344, 11.0832) (-4.5292, 11.0579) (-4.5237, 11.0327) (-4.5181, 11.0076) (-4.5124, 10.9825) (-4.5064, 10.9575) (-4.5, 10.9327) (-4.4929, 10.9081) (-4.4865, 10.8887) (-4.4812, 10.8743) (-4.4774, 10.8648) (-4.4755, 10.8601) knots -1 -1 -1 -1 -1 -1 -0.98571429 -0.97142857 -0.95714286 -0.94285714 -0.92857143 -0.91428571 -0.9 -0.88571429 -0.87142857 -0.85714286 -0.84285714 -0.82857143 -0.81428571 -0.8 -0.78571429 -0.77142857 -0.75714286 -0.74285714 -0.72857143 -0.71428571 -0.7 -0.68571429 -0.67142857 -0.65714286 -0.64285714 -0.62857143 -0.61428571 -0.6 -0.58571429 -0.57142857 -0.55714286 -0.54285714 -0.52857143 -0.51428571 -0.5 -0.48571429 -0.47142857 -0.45714286 -0.44285714 -0.42857143 -0.41428571 -0.4 -0.38571429 -0.37142857 -0.35714286 -0.34285714 -0.32857143 -0.31428571 -0.3 -0.28571429 -0.27142857 -0.25714286 -0.24285714 -0.22857143 -0.21428571 -0.2 -0.18571429 -0.17142857 -0.15714286 -0.14285714 -0.12857143 -0.11428571 -0.1 -0.08571429 -0.07142857 -0.05714286 -0.04285714 -0.02857143 -0.01428571 0 0 0 0 0 0
  line L41 (-4.4755, 10.8601) -> (-4.4347, 10.7612)
  arc A83 (-4.5907, 10.3725) -> (-4.4347, 10.7612) centre (-4.7121, 10.6469) ccw
  arc A84 (-4.5907, 10.3725) -> (-5.066, 10.1489) centre (0, 0) ccw
  arc A85 (-5.4648, 10.2764) -> (-5.066, 10.1489) centre (-5.2, 10.4173) ccw
  line L42 (-5.4648, 10.2764) -> (-5.5151, 10.3709)
  spline S42 degree 5 poles (-5.5151, 10.3709) (-5.5175, 10.3754) (-5.5224, 10.3844) (-5.5301, 10.3976) (-5.5409, 10.4149) (-5.5554, 10.436) (-5.5704, 10.4568) (-5.5859, 10.4773) (-5.6015, 10.4978) (-5.6173, 10.5181) (-5.6332, 10.5384) (-5.6494, 10.5585) (-5.6657, 10.5785) (-5.6824, 10.5983) (-5.6994, 10.618) (-5.7166, 10.6375) (-5.7341, 10.6568) (-5.7517, 10.676) (-5.7696, 10.6951) (-5.7876, 10.7141) (-5.8057, 10.733) (-5.8241, 10.7518) (-5.8426, 10.7704) (-5.8612, 10.789) (-5.8801, 10.8074) (-5.8991, 10.8257) (-5.9183, 10.844) (-5.9377, 10.8621) (-5.9572, 10.8801) (-5.9768, 10.898) (-5.9966, 10.9158) (-6.0165, 10.9335) (-6.0366, 10.9511) (-6.0568, 10.9687) (-6.0772, 10.9861) (-6.0977, 11.0034) (-6.1183, 11.0206) (-6.1391, 11.0377) (-6.16, 11.0548) (-6.181, 11.0717) (-6.2022, 11.0885) (-6.2234, 11.1053) (-6.2448, 11.122) (-6.2664, 11.1385) (-6.288, 11.155) (-6.3098, 11.1714) (-6.3316, 11.1877) (-6.3537, 11.2039) (-6.3758, 11.22) (-6.398, 11.236) (-6.4203, 11.2519) (-6.4428, 11.2678) (-6.4654, 11.2835) (-6.4881, 11.2992) (-6.5109, 11.3148) (-6.5338, 11.3303) (-6.5568, 11.3457) (-6.5799, 11.361) (-6.6031, 11.3762) (-6.6264, 11.3914) (-6.6499, 11.4064) (-6.6734, 11.4214) (-6.697, 11.4363) (-6.7208, 11.451) (-6.7446, 11.4658) (-6.7685, 11.4804) (-6.7926, 11.4949) (-6.8167, 11.5094) (-6.8409, 11.5237) (-6.8653, 11.538) (-6.8897, 11.5522) (-6.9093, 11.5635) (-6.924, 11.5719) (-6.9339, 11.5775) (-6.9388, 11.5803) knots 0 0 0 0 0 0 0.01428571 0.02857143 0.04285714 0.05714286 0.07142857 0.08571429 0.1 0.11428571 0.12857143 0.14285714 0.15714286 0.17142857 0.18571429 0.2 0.21428571 0.22857143 0.24285714 0.25714286 0.27142857 0.28571429 0.3 0.31428571 0.32857143 0.34285714 0.35714286 0.37142857 0.38571429 0.4 0.41428571 0.42857143 0.44285714 0.45714286 0.47142857 0.48571429 0.5 0.51428571 0.52857143 0.54285714 0.55714286 0.57142857 0.58571429 0.6 0.61428571 0.62857143 0.64285714 0.65714286 0.67142857 0.68571429 0.7 0.71428571 0.72857143 0.74285714 0.75714286 0.77142857 0.78571429 0.8 0.81428571 0.82857143 0.84285714 0.85714286 0.87142857 0.88571429 0.9 0.91428571 0.92857143 0.94285714 0.95714286 0.97142857 0.98571429 1 1 1 1 1 1
  arc A86 (-6.9388, 11.5803) -> (-7.5237, 11.2091) centre (0, 0) ccw
  spline S43 degree 5 poles (-7.5237, 11.2091) (-7.5233, 11.2034) (-7.5224, 11.1921) (-7.5211, 11.1752) (-7.5192, 11.1526) (-7.5168, 11.1245) (-7.5142, 11.0964) (-7.5116, 11.0684) (-7.5088, 11.0404) (-7.5059, 11.0125) (-7.5028, 10.9846) (-7.4997, 10.9567) (-7.4964, 10.929) (-7.493, 10.9012) (-7.4895, 10.8736) (-7.4858, 10.846) (-7.4821, 10.8184) (-7.4782, 10.7909) (-7.4741, 10.7635) (-7.47, 10.7361) (-7.4657, 10.7088) (-7.4614, 10.6815) (-7.4568, 10.6544) (-7.4522, 10.6272) (-7.4474, 10.6002) (-7.4425, 10.5731) (-7.4375, 10.5462) (-7.4323, 10.5193) (-7.427, 10.4925) (-7.4216, 10.4658) (-7.416, 10.4391) (-7.4104, 10.4125) (-7.4045, 10.386) (-7.3986, 10.3595) (-7.3925, 10.3332) (-7.3862, 10.3068) (-7.3799, 10.2806) (-7.3733, 10.2545) (-7.3667, 10.2284) (-7.3599, 10.2024) (-7.3529, 10.1765) (-7.3459, 10.1506) (-7.3386, 10.1249) (-7.3312, 10.0992) (-7.3237, 10.0736) (-7.316, 10.0481) (-7.3081, 10.0227) (-7.3002, 9.9974) (-7.292, 9.9722) (-7.2837, 9.9471) (-7.2752, 9.9221) (-7.2666, 9.8971) (-7.2577, 9.8723) (-7.2487, 9.8476) (-7.2395, 9.8231) (-7.2302, 9.7986) (-7.2206, 9.7742) (-7.2109, 9.7499) (-7.2011, 9.7258) (-7.191, 9.7017) (-7.1808, 9.6778) (-7.1702, 9.6541) (-7.1594, 9.6306) (-7.1482, 9.6073) (-7.1369, 9.5841) (-7.1253, 9.5611) (-7.1136, 9.5381) (-7.1018, 9.5153) (-7.0898, 9.4926) (-7.0775, 9.4701) (-7.0645, 9.4481) (-7.0535, 9.4309) (-7.0448, 9.4183) (-7.0387, 9.41) (-7.0357, 9.4059) knots -1 -1 -1 -1 -1 -1 -0.98571429 -0.97142857 -0.95714286 -0.94285714 -0.92857143 -0.91428571 -0.9 -0.88571429 -0.87142857 -0.85714286 -0.84285714 -0.82857143 -0.81428571 -0.8 -0.78571429 -0.77142857 -0.75714286 -0.74285714 -0.72857143 -0.71428571 -0.7 -0.68571429 -0.67142857 -0.65714286 -0.64285714 -0.62857143 -0.61428571 -0.6 -0.58571429 -0.57142857 -0.55714286 -0.54285714 -0.52857143 -0.51428571 -0.5 -0.48571429 -0.47142857 -0.45714286 -0.44285714 -0.42857143 -0.41428571 -0.4 -0.38571429 -0.37142857 -0.35714286 -0.34285714 -0.32857143 -0.31428571 -0.3 -0.28571429 -0.27142857 -0.25714286 -0.24285714 -0.22857143 -0.21428571 -0.2 -0.18571429 -0.17142857 -0.15714286 -0.14285714 -0.12857143 -0.11428571 -0.1 -0.08571429 -0.07142857 -0.05714286 -0.04285714 -0.02857143 -0.01428571 0 0 0 0 0 0
  line L43 (-7.0357, 9.4059) -> (-6.9716, 9.3202)
  arc A87 (-7.026, 8.905) -> (-6.9716, 9.3202) centre (-7.2118, 9.1405) ccw
  arc A88 (-7.026, 8.905) -> (-7.4307, 8.5702) centre (0, 0) ccw
  arc A89 (-7.8488, 8.5945) -> (-7.4307, 8.5702) centre (-7.6273, 8.7968) ccw
  line L44 (-7.8488, 8.5945) -> (-7.921, 8.6736)